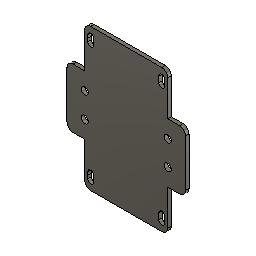
spindle-mount-adapter-plate (Autodesk Fusion 360 design; units mm, degrees)
Autodesk Fusion 360 part; units mm, degrees
note: some values were not read from the file. Set by a fixed rule: which sketch regions a step uses.
sketch "Sketch1" plane through (0, 0, 0) normal (0, 0, 1) x (1, 0, 0)
  line L0 (30, 50) -> (-30, 50)
  line L1 (-30, 50) -> (-30, -50)
  line L2 (-30, -50) -> (30, -50)
  line L3 (30, -50) -> (30, 50)
  line L4 (30, 50) -> (-30, -50) construction
  line L5 (-30, 50) -> (30, -50) construction
  line L6 (45, 25) -> (-45, 25)
  line L7 (-50, 20) -> (-50, -20)
  line L8 (-45, -25) -> (45, -25)
  line L9 (50, -20) -> (50, 20)
  line L10 (50, 25) -> (-50, -25) construction
  line L11 (-50, 25) -> (50, -25) construction
  line L12 (35, 10.5) -> (-35, 10.5) construction
  line L13 (-35, 10.5) -> (-35, -10.5) construction
  line L14 (-35, -10.5) -> (35, -10.5) construction
  line L15 (35, -10.5) -> (35, 10.5) construction
  line L16 (35, 10.5) -> (-35, -10.5) construction
  line L17 (-35, 10.5) -> (35, -10.5) construction
  circle A0 centre (-35, 10.5) radius 3
  circle A1 centre (-35, -10.5) radius 3
  circle A2 centre (35, 10.5) radius 3
  circle A3 centre (35, -10.5) radius 3
  line L18 (-27.5, 47.5) -> (-27.5, 52.5)
  arc A4 (-27.5, 52.5) -> (-32.5, 52.5) centre (-30, 52.5) ccw
  line L19 (-32.5, 52.5) -> (-32.5, 47.5)
  arc A5 (-32.5, 47.5) -> (-27.5, 47.5) centre (-30, 47.5) ccw
  line L20 (-30, 47.5) -> (-30, 52.5) construction
  line L21 (32.5, 47.5) -> (32.5, 52.5)
  arc A6 (32.5, 52.5) -> (27.5, 52.5) centre (30, 52.5) ccw
  line L22 (27.5, 52.5) -> (27.5, 47.5)
  arc A7 (27.5, 47.5) -> (32.5, 47.5) centre (30, 47.5) ccw
  line L23 (30, 47.5) -> (30, 52.5) construction
  line L24 (-70, 0) -> (55, 0) construction
  arc A8 (-32.5, -52.5) -> (-27.5, -52.5) centre (-30, -52.5) ccw
  line L25 (-32.5, -52.5) -> (-32.5, -47.5)
  line L26 (-27.5, -47.5) -> (-27.5, -52.5)
  arc A9 (-27.5, -47.5) -> (-32.5, -47.5) centre (-30, -47.5) ccw
  arc A10 (32.5, -47.5) -> (27.5, -47.5) centre (30, -47.5) ccw
  arc A11 (27.5, -52.5) -> (32.5, -52.5) centre (30, -52.5) ccw
  line L27 (27.5, -52.5) -> (27.5, -47.5)
  line L28 (32.5, -47.5) -> (32.5, -52.5)
  line L29 (30, 60) -> (-30, 60)
  line L30 (-35, 55) -> (-35, -55)
  line L31 (-30, -60) -> (30, -60)
  line L32 (35, -55) -> (35, 55)
  line L33 (35, 60) -> (-35, -60) construction
  line L34 (-35, 60) -> (35, -60) construction
  arc A12 (-30, 60) -> (-35, 55) centre (-30, 55) ccw
  arc A13 (35, 55) -> (30, 60) centre (30, 55) ccw
  arc A14 (-35, -55) -> (-30, -60) centre (-30, -55) ccw
  arc A15 (30, -60) -> (35, -55) centre (30, -55) ccw
  arc A16 (-27.5, -50.0014) -> (-27.5, -49.9986) centre (-30, -50) ccw
  arc A17 (-32.5, -49.9986) -> (-32.5, -50.0014) centre (-30, -50) ccw
  arc A18 (-32.5, 50.0024) -> (-32.5, 49.9976) centre (-30, 50) ccw
  arc A19 (-27.5, 50) -> (-27.5, 50.0014) centre (-30, 50) ccw
  arc A20 (50, 20) -> (45, 25) centre (45, 20) ccw
  arc A21 (45, -25) -> (50, -20) centre (45, -20) ccw
  arc A22 (-50, -20) -> (-45, -25) centre (-45, -20) ccw
  arc A23 (-45, 25) -> (-50, 20) centre (-45, 20) ccw
  point P0 (-30, 50)
  point P1 (30, 50)
  dimension "d1" = 60
  dimension "d2" = 100
  dimension "d5" = 5
  dimension "d7" = 100
  dimension "d8" = 50
  dimension "d9" = 70
  dimension "d10" = 21
  dimension "d12" = 6
  dimension "d13" = 6
  dimension "d14" = 6
  dimension "d15" = 6
  dimension "d16" = 5
  dimension "d17" = 70
  dimension "d18" = 120
  dimension "d19" = 5
  dimension "d20" = 5
  constraint horizontal L0
  constraint perpendicular L0 L1
  constraint parallel L0 L2
  constraint parallel L1 L3
  constraint coincident L4 origin
  constraint coincident L5 origin
  constraint coincident L1.end L2.start
  constraint horizontal L6
  constraint perpendicular L6 L7
  constraint parallel L6 L8
  constraint parallel L7 L9
  constraint coincident L10 origin
  constraint coincident L11 origin
  constraint horizontal L12
  constraint perpendicular L12 L13
  constraint parallel L12 L14
  constraint parallel L13 L15
  constraint coincident L16 origin
  constraint coincident L17 origin
  constraint coincident L12.end L13.start
  constraint coincident L13.end L14.start
  constraint coincident L12.start L15.end
  constraint coincident L14.end L15.start
  constraint tangent L18 A4
  constraint tangent A4 L19
  constraint parallel L18 L19
  constraint tangent L19 A5
  constraint tangent L18 A5
  constraint perpendicular L0 L20
  constraint midpoint L20 P0
  constraint tangent L21 A6
  constraint tangent A6 L22
  constraint parallel L21 L22
  constraint tangent L22 A7
  constraint tangent L21 A7
  constraint parallel L3 L23
  constraint midpoint L23 P1
  constraint perpendicular L9 L24
  constraint symmetric L18.start L24 L26.start
  constraint symmetric L18.end L24 A8.end
  constraint symmetric A4.end L24 A8.start
  constraint symmetric L19.end L24 L25.end
  constraint symmetric A4 L24 A8
  constraint symmetric A5 L24 A9
  constraint symmetric L21.start L24 A10.start
  constraint symmetric L21.end L24 A11.end
  constraint symmetric A6.end L24 A11.start
  constraint symmetric L22.end L24 A10.end
  constraint symmetric A6 L24 A11
  constraint symmetric A7 L24 A10
  constraint horizontal L29
  constraint perpendicular L29 L30
  constraint parallel L29 L31
  constraint parallel L30 L32
  constraint coincident L33 origin
  constraint coincident L34 origin
  constraint coincident L34.start L30
  constraint coincident L34.start L29
  constraint tangent L30 A12
  constraint tangent L29 A12
  constraint coincident L33.start L29
  constraint coincident L33.start L32
  constraint tangent L29 A13
  constraint tangent L32 A13
  constraint equal A12 A13
  constraint coincident L33.end L30
  constraint coincident L33.end L31
  constraint tangent L30 A14
  constraint tangent L31 A14
  constraint equal A12 A14
  constraint coincident L34.end L31
  constraint coincident L34.end L32
  constraint tangent L31 A15
  constraint tangent L32 A15
  constraint equal A12 A15
  constraint coincident L25 A17.end
  constraint coincident L25 A17.start
  constraint concentric A16 A17
  constraint coincident L26 A16.end
  constraint coincident L26 A16.start
  constraint coincident L18 A19.end
  constraint coincident L19 A18.start
  constraint coincident L19 A18.end
  constraint coincident L0 A19.start
  constraint coincident L10.start L6
  constraint coincident L10.start L9
  constraint tangent L6 A20
  constraint tangent L9 A20
  constraint coincident L11.end L8
  constraint coincident L11.end L9
  constraint tangent L8 A21
  constraint tangent L9 A21
  constraint equal A20 A21
  constraint coincident L10.end L8
  constraint coincident L10.end L7
  constraint tangent L8 A22
  constraint tangent L7 A22
  constraint equal A20 A22
  constraint coincident L11.start L7
  constraint coincident L11.start L6
  constraint tangent L7 A23
  constraint tangent L6 A23
  constraint equal A20 A23
  measures "d1" distance of L1.end L2.end
  measures "d2" distance of P0 L1.end
  measures "d5" diameter of A16
  measures "d7" distance of L10.end L11.end
  measures "d8" distance of L11.start L10.end
  measures "d9" distance of L13.end L14.end
  measures "d10" distance of L12.end L13.end
  measures "d12" diameter of A0
  measures "d13" diameter of A1
  measures "d14" diameter of A2
  measures "d15" diameter of A3
  measures "d16" diameter of A6
  measures "d17" distance of L33.start L34.start
  measures "d18" distance of L33.start L34.end
  measures "d19" radius of A12
  measures "d20" radius of A20
extrude "Extrude1" add sketch "Sketch1" along normal blind 3 contours L0 L1 L3 L6 L18 A4 L19 A5 L21 A6 L22 A7 L29 L30 L32 A12 A13 A18 A19 | L0 L1 L3 L6 L18 A5 L22 A7 | L1 L3 L6 L8 | L1 L6 L8 A0 A1 L30 | L3 L6 L8 A2 A3 L32 | L1 L2 L3 L8 L26 A9 A10 L27 | L1 L2 L3 L8 A8 L25 L26 A9 A10 A11 L27 L28 L30 L31 L32 A14 A15 A17 | L6 L7 L8 A0 A1 L30 A22 A23 | L6 L8 L9 A2 A3 L32 A20 A21
sketch "dfx_export" plane through (0, 0, 3) normal (0, 0, 1) x (1, 0, 0)
  arc A0 (-27.5, -47.5) -> (-32.5, -47.5) centre (-30, -47.5) ccw
  line L0 (-27.5, -47.5) -> (-27.5, -49.9986)
  arc A1 (-27.5, -50.0014) -> (-27.5, -49.9986) centre (-30, -50) ccw
  line L1 (-27.5, -50.0014) -> (-27.5, -52.5)
  arc A2 (-32.5, -52.5) -> (-27.5, -52.5) centre (-30, -52.5) ccw
  line L2 (-32.5, -52.5) -> (-32.5, -50.0014)
  arc A3 (-32.5, -49.9986) -> (-32.5, -50.0014) centre (-30, -50) ccw
  line L3 (-32.5, -49.9986) -> (-32.5, -47.5)
  arc A4 (27.5, 47.5) -> (32.5, 47.5) centre (30, 47.5) ccw
  line L4 (27.5, 47.5) -> (27.5, 52.5)
  arc A5 (32.5, 52.5) -> (27.5, 52.5) centre (30, 52.5) ccw
  line L5 (32.5, 52.5) -> (32.5, 47.5)
  arc A6 (-27.5, 50) -> (-27.5, 50.0014) centre (-30, 50) ccw
  line L6 (-27.5, 50) -> (-27.5, 47.5)
  arc A7 (-32.5, 47.5) -> (-27.5, 47.5) centre (-30, 47.5) ccw
  line L7 (-32.5, 47.5) -> (-32.5, 49.9976)
  arc A8 (-32.5, 50.0024) -> (-32.5, 49.9976) centre (-30, 50) ccw
  line L8 (-32.5, 50.0024) -> (-32.5, 52.5)
  arc A9 (-27.5, 52.5) -> (-32.5, 52.5) centre (-30, 52.5) ccw
  line L9 (-27.5, 52.5) -> (-27.5, 50.0014)
  arc A10 (27.5, -52.5) -> (32.5, -52.5) centre (30, -52.5) ccw
  line L10 (27.5, -52.5) -> (27.5, -47.5)
  arc A11 (32.5, -47.5) -> (27.5, -47.5) centre (30, -47.5) ccw
  line L11 (32.5, -47.5) -> (32.5, -52.5)
  circle A12 centre (35, -10.5) radius 3
  circle A13 centre (35, 10.5) radius 3
  circle A14 centre (-35, 10.5) radius 3
  circle A15 centre (-35, -10.5) radius 3
  arc A16 (-45, 25) -> (-50, 20) centre (-45, 20) ccw
  line L12 (-50, 20) -> (-50, -20)
  arc A17 (-50, -20) -> (-45, -25) centre (-45, -20) ccw
  line L13 (-45, -25) -> (-35, -25)
  line L14 (-35, -25) -> (-35, -55)
  arc A18 (-35, -55) -> (-30, -60) centre (-30, -55) ccw
  line L15 (-30, -60) -> (30, -60)
  arc A19 (30, -60) -> (35, -55) centre (30, -55) ccw
  line L16 (35, -55) -> (35, -25)
  line L17 (35, -25) -> (45, -25)
  arc A20 (45, -25) -> (50, -20) centre (45, -20) ccw
  line L18 (50, -20) -> (50, 20)
  arc A21 (50, 20) -> (45, 25) centre (45, 20) ccw
  line L19 (45, 25) -> (35, 25)
  line L20 (35, 25) -> (35, 55)
  arc A22 (35, 55) -> (30, 60) centre (30, 55) ccw
  line L21 (30, 60) -> (-30, 60)
  arc A23 (-30, 60) -> (-35, 55) centre (-30, 55) ccw
  line L22 (-35, 55) -> (-35, 25)
  line L23 (-35, 25) -> (-45, 25)
